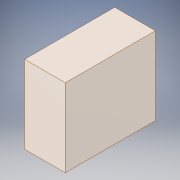
# Autodesk Inventor part: KST DS215MG V3
Saved by Autodesk Inventor 2018.2 (Build 222227000, 227)
## iProperties
Created: 2014-12-10
Part Number: KST DS215MG V3
Material: SolidWorks Materials|ABS|33
Document SubType Name: Modeling
Designer: JochenAlt
Density: 1.02 g/cm^3
Appearance: 192,192,192
Sending System: SolidWorks 2014
Last Author: Main
Last Saved: 2014-12-10
Author: JochenAlt
Autodesk Inventor part; units mm, degrees
ref_plane "YZ Plane" through (0, 0, 0) normal (1, 0, 0) x (0, 1, 0)
ref_plane "XY Plane" through (0, 0, 0) normal (0, 0, 1) x (1, 0, 0)
feature "Spline" [suppressed]
ref_plane "Arbeitsebene1" through (0, -4.5, 0) normal (0, 1, 0) x (-1, 0, 0)
sketch "Skizze1" plane through (0, -4.5, 0) normal (0, 1, 0) x (-1, 0, 0)
  line L0 (-11.816, -0.5855) -> (-11.816, -23.5855)
  line L1 (0.184, -23.5855) -> (0.184, -0.5855)
  circle A0 centre (-5.816, -17.7855) radius 1 construction
  line L2 (-5.816, 7.3911) -> (-5.816, -23.5855) construction
  line L3 (0.184, -0.5855) -> (-11.816, -0.5855)
  line L4 (-11.816, -0.5855) -> (-11.816, 3.9145)
  line L5 (0.184, 3.9145) -> (0.184, -0.5855)
  line L6 (0.184, -23.5855) -> (-11.816, -23.5855)
  line L7 (-11.816, -23.5855) -> (-11.816, -28.0855)
  line L8 (0.184, -28.0855) -> (0.184, -23.5855)
  circle A1 centre (-2.316, -26.0855) radius 1.3
  circle A2 centre (-9.316, -26.0855) radius 1.3
  circle A3 centre (-2.316, 1.9145) radius 1.3
  circle A4 centre (-9.316, 1.9145) radius 1.3
  line L9 (-2.316, 1.9145) -> (-2.316, -26.0855) construction
  line L10 (-2.316, -26.0855) -> (-9.316, -26.0855) construction
  line L11 (-9.316, -26.0855) -> (-9.316, 1.9145) construction
  line L12 (-9.316, 1.9145) -> (-2.316, 1.9145) construction
  arc A5 (-6.816, 1.9145) -> (-4.816, 1.9145) centre (-5.816, 1.9145) ccw
  arc A6 (-4.816, -26.0855) -> (-6.816, -26.0855) centre (-5.816, -26.0855) ccw
  line L13 (-4.816, 1.9145) -> (-4.816, 3.9145)
  line L14 (-6.816, 1.9145) -> (-6.816, 3.9145)
  line L15 (-4.816, -26.0855) -> (-4.816, -28.0855)
  line L16 (-6.816, -26.0855) -> (-6.816, -28.0855)
  line L17 (-11.816, -28.0855) -> (-6.816, -28.0855)
  line L18 (-4.816, -28.0855) -> (0.184, -28.0855)
  line L19 (-11.816, 3.9145) -> (-6.816, 3.9145)
  line L20 (-4.816, 3.9145) -> (0.184, 3.9145)
  point P0 (0, 0)
  point P1 (-5.816, -26.0855)
  dimension "d1" = 5.8
  dimension "d2" = 12
  dimension "d3" = 7
  dimension "d4" = 8.3
  dimension "d5" = 2.6
  dimension "d6" = 28
  dimension "d7" = 32
  dimension "d8" = 23
  dimension "d9" = 1
  constraints: 42 end point, 11 parallel, 6 centre point, 4 collinear, 4 equal radius, 4 point on circle, 4 tangent, 4 vertical, 3 perpendicular, 2 horizontal, 2 midpoint, 1 coincident, 1 point on line, 3 other
  measures "d1" distance from line of L6 A0.centre
  measures "d2" distance between parallel lines of L7 L8
  measures "d3" distance between parallel lines of L11 L9
  measures "d4" distance from line of L10 A0.centre
  measures "d5" diameter of A1
  measures "d6" distance of L9.start L9.end
  measures "d7" distance between parallel lines of L18 L20
  measures "d8" distance between parallel lines of L6 L3
  measures "d9" radius of A6
extrude "Extrusion1" add sketch "Skizze1" along normal blind 26.6 contours L3 L1 L6 L0
ref_plane "Arbeitsebene3" through (0, 16.6, 0) normal (0, 1, 0) x (-1, 0, 0)
sketch "Skizze2" plane through (0, 16.6, 0) normal (0, 1, 0) x (-1, 0, 0)
  line L0 (-4.816, 3.9145) -> (0.184, 3.9145) projected
  line L1 (0.184, 3.9145) -> (0.184, -0.5855) projected
  line L2 (-4.816, 1.9145) -> (-4.816, 3.9145) projected
  arc A0 (-6.816, 1.9145) -> (-4.816, 1.9145) centre (-5.816, 1.9145) ccw projected
  line L3 (-6.816, 1.9145) -> (-6.816, 3.9145) projected
  line L4 (-11.816, 3.9145) -> (-6.816, 3.9145) projected
  circle A1 centre (-9.316, 1.9145) radius 1.3 projected
  circle A2 centre (-2.316, 1.9145) radius 1.3 projected
  line L5 (-11.816, -0.5855) -> (-11.816, 3.9145) projected
  line L6 (0.184, -0.5855) -> (-11.816, -0.5855) projected
  line L7 (-11.816, -23.5855) -> (0.184, -23.5855) projected
  line L8 (0.184, -28.0855) -> (0.184, -23.5855) projected
  line L9 (-4.816, -28.0855) -> (0.184, -28.0855) projected
  circle A3 centre (-2.316, -26.0855) radius 1.3 projected
  line L10 (-4.816, -26.0855) -> (-4.816, -28.0855) projected
  arc A4 (-4.816, -26.0855) -> (-6.816, -26.0855) centre (-5.816, -26.0855) ccw projected
  line L11 (-6.816, -26.0855) -> (-6.816, -28.0855) projected
  line L12 (-11.816, -28.0855) -> (-6.816, -28.0855) projected
  circle A5 centre (-9.316, -26.0855) radius 1.3 projected
  line L13 (-11.816, -23.5855) -> (-11.816, -28.0855) projected
  line L14 (0.184, -0.5855) -> (-11.816, -0.5855) projected
  line L15 (-11.816, -0.5855) -> (-11.816, -23.5855) projected
  line L16 (-11.816, -23.5855) -> (0.184, -23.5855) projected
  line L17 (0.184, -23.5855) -> (0.184, -0.5855) projected
  point P0 (0, 0)
extrude "Extrusion2" [suppressed]
sketch "Skizze4" plane through (11.816, -4.5, -23.5855) normal (0, 0, -1) x (-1, 0, 0)
  line L0 (4.5, 7.75) -> (7.5, 7.75)
  line L1 (7.5, 7.75) -> (7.5, 6.25)
  line L2 (7.5, 6.25) -> (4.5, 6.25)
  line L3 (4.5, 6.25) -> (4.5, 7.75)
  line L4 (4.5, 7) -> (7.5, 7) construction
  line L5 (0, 0) -> (0, 26.6) construction
  line L6 (0, 0) -> (12, 0) construction
  line L7 (12, 0) -> (12, 26.6) construction
  line L8 (6, 7.75) -> (6, 6.25) construction
  line L9 (0, 26.6) -> (12, 26.6) projected
  point P0 (11.816, 4.5)
  dimension "d19" = 7
  dimension "d20" = 1.5
  dimension "d21" = 4.5
  dimension "d22" = 4.5
  constraints: 12 end point, 4 midpoint, 2 parallel, 1 horizontal, 1 perpendicular
  measures "d19" distance between parallel lines of L6 L4
  measures "d20" distance between parallel lines of L2 L0
  measures "d21" distance between parallel lines of L5 L3
  measures "d22" distance between parallel lines of L7 L1
extrude "Extrusion3" [suppressed]
fillet "Rundung2" [suppressed]
fillet "Rundung1" [suppressed]
equation "\"d22\" = d21"
